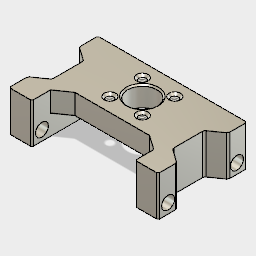
Z_Trapezoidal_Nut_Holder_Upgrade (Autodesk Fusion 360 design; units mm, degrees)
Autodesk Fusion 360 part; units mm, degrees
sketch "Sketch1" plane through (0, 0, 0) normal (0, 1, 0) x (1, 0, 0)
  circle A0 centre (0, 0) radius 5.1
  circle A1 centre (5.6569, 5.6569) radius 1.5
  circle A2 centre (-5.6569, 5.6569) radius 1.5
  circle A3 centre (-5.6569, -5.6569) radius 1.5
  circle A4 centre (5.6569, -5.6569) radius 1.5
  line L0 (0, 0) -> (0, -5) construction
  line L1 (0, -5) -> (21, -5) construction
  line L2 (21, -5) -> (21, 0.5)
  line L3 (21, 0.5) -> (26, 4)
  line L4 (26, 4) -> (26, 10.5)
  line L5 (26, -14) -> (26, -20.5)
  line L6 (21, -10.5) -> (26, -14)
  line L7 (21, -5) -> (21, -10.5)
  line L8 (-26, 4) -> (-26, 10.5)
  line L9 (-21, 0.5) -> (-26, 4)
  line L10 (-21, -5) -> (-21, 0.5)
  line L11 (-21, -5) -> (-21, -10.5)
  line L12 (-21, -10.5) -> (-26, -14)
  line L13 (-26, -14) -> (-26, -20.5)
  line L14 (0, -5) -> (-21, -5) construction
  line L15 (-26, -20.5) -> (-18, -20.5)
  line L16 (-18, -20.5) -> (-18, -14)
  line L17 (-18, -14) -> (-13, -10.5)
  line L18 (18, -14) -> (13, -10.5)
  line L19 (18, -20.5) -> (18, -14)
  line L20 (26, -20.5) -> (18, -20.5)
  line L21 (13, -10.5) -> (-13, -10.5)
  line L22 (26, 10.5) -> (-26, 10.5)
  line L23 (-18, -14) -> (-18, 10.5)
  line L24 (18, -14) -> (18, 10.5)
  dimension "d1" = 10.2
  dimension "d2" = 3
  dimension "d4" = 360
  dimension "d5" = 16
  dimension "d22" = 5
  dimension "d24" = 5.5
  dimension "d25" = 5
  dimension "d26" = 6.5
  dimension "d27" = 31
  dimension "d28" = 52
  dimension "d31" = 21
  dimension "d32" = 8
  measures "d1" diameter of A0
  measures "d2" diameter of A1
  measures "d5" distance of A1.centre A3.centre
  measures "d22" distance of A0.centre L0.end
  measures "d24" distance of L1.end L2.end
  measures "d25" distance of L2 L4
  measures "d26" distance of L3.end L4.end
  measures "d27" distance of L4.end L5.end
  measures "d28" distance of L5 L13
  measures "d31" distance of L21 L22
  measures "d32" distance of L13.end L15.end
extrude "Extrude1" add sketch "Sketch1" against normal blind 14 contours L2 L3 L4 L5 L6 L7 L19 L20 L22 L24 | L8 L9 L10 L11 L12 L13 L15 L16 L22 L23 makes body 1 at (-18, -4.6667, 10.1667) makes body 2 at (18, -9.3333, -0.1667)
extrude "Extrude2" add sketch "Sketch1" against normal blind 7 contours L17 L18 L21 L22 L23 L24 bodies 1 2
sketch "Sketch2" plane through (26, 0, 0) normal (1, 0, 0) x (0, 0, -1)
  line L0 (10.5, 0) -> (4, 0)
  line L1 (4, 0) -> (4, -14)
  line L2 (4, -14) -> (10.5, -14)
  line L3 (10.5, -14) -> (10.5, 0)
  line L4 (-20.5, -14) -> (10.5, -14)
  line L5 (-20.5, 0) -> (-14, 0)
  circle A0 centre (7, -10.5) radius 2.25
  circle A1 centre (-17, -10.5) radius 2.25
  dimension "d37" = 4.5
  dimension "d38" = 4.5
  dimension "d43" = 24
  dimension "d44" = 3.5
  measures "d37" diameter of A0
  measures "d38" diameter of A1
  measures "d43" distance of A0.centre A1.centre
  measures "d44" distance of L3 A0.centre
extrude "Extrude3" cut sketch "Sketch2" against normal through all contours A0 | A1 bodies 1
chamfer "Chamfer1" distance 0.5 angle 45 15 edges at (-4.7549, 0, 1.8442) (-7.0553, 0, -5.1144) (4.2584, 0, -5.1144) (4.2584, 0, 6.1993) (-7.0553, 0, 6.1993) (26, -7, -10.5) (26, -7, -4) (26, -7, 14) (26, -7, 20.5) (18, -7, 20.5) (-18, -7, 20.5) (-26, -7, 20.5) (-26, -7, 14) (-26, -7, -4) (-26, -7, -10.5) on bodies 1
fillet "Fillet2" radius 1 4 edges at (21, -7, -0.5) (21, -7, 10.5) (-21, -7, 10.5) (-21, -7, -0.5) on bodies 1
thread "Thread1" "ISO Metric profile 3.0 M3x0.5 6H" major diameter 3.086 minor diameter 2.529 pitch 0.5 angle 60 resizes the face on face at (-4.1643, -2.6667, 5.8062) on face at (-4.1643, -2.6667, -5.5075) on face at (7.1494, -2.6667, -5.5075) on face at (7.1494, -2.6667, 5.8062) on bodies 1
